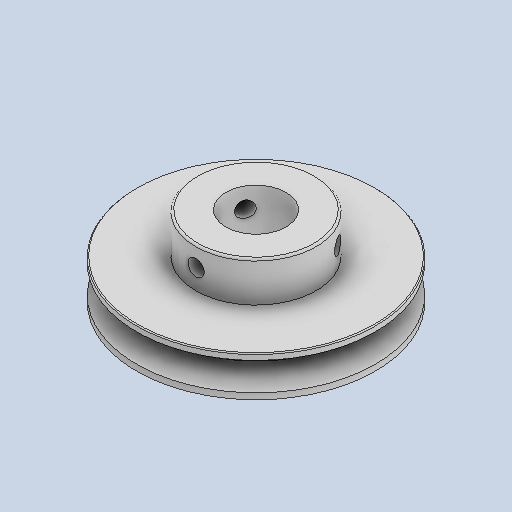
# Autodesk Inventor part: Шкив 119 мм
Saved by Autodesk Inventor 2025 (Build 290162010, 162A)
## iProperties
Created: 2024-04-08
Part Number: Шкив 119 мм
Material: Generic
Document SubType Name: Modeling
Designer: pokla
Density: 1 g/cm^3
Appearance: Default
Author: pokla
Autodesk Inventor part; units mm, degrees
ref_plane "YZ Plane" through (0, 0, 0) normal (1, 0, 0) x (0, 1, 0)
ref_plane "XZ Plane" through (0, 0, 0) normal (0, 1, 0) x (-1, 0, 0)
ref_plane "XY Plane" through (0, 0, 0) normal (0, 0, 1) x (1, 0, 0)
sketch "Sketch1" plane through (0, 0, 0) normal (1, 0, 0) x (0, 1, 0)
  line L0 (0, -15) -> (40, -15)
  line L1 (40, -15) -> (40, -30)
  line L2 (40, -30) -> (20, -30)
  line L3 (20, -30) -> (20, -59.5)
  line L4 (20, -59.5) -> (17, -59.5)
  line L5 (17, -59.5) -> (12.5, -46.5)
  line L6 (12.5, -46.5) -> (7.5, -46.5)
  line L7 (3, -59.5) -> (0, -59.5)
  line L8 (0, -59.5) -> (0, -15)
  line L9 (7.5, -46.5) -> (3, -59.5)
  line L10 (-8, 0) -> (48, 0) projected
  point P0 (0, 0)
  point P1 (0, -37.25)
  dimension "d0" = 15
  dimension "d1" = 59.5
  dimension "d2" = 40
  dimension "d3" = 20
  dimension "d4" = 5
  dimension "d5" = 3
  dimension "d7" = 46.5
  dimension "d8" = 15
  constraints: 20 end point, 5 perpendicular, 2 equal length, 2 point on line, 1 horizontal, 1 midpoint, 1 parallel, 1 vertical alignment
  measures "d0" distance of point (0, 0) L0.start
  measures "d1" distance of L7.end point (0, 0)
  measures "d2" distance of L0.start L0.end
  measures "d3" distance between parallel lines of L8 L3
  measures "d4" distance of L5.end L6.end
  measures "d5" distance of L7.start L7.end
  measures "d7" distance from line of point (0, 0) L6
  measures "d8" distance of L0.end L1.end
revolve "Revolution1" add sketch "Sketch1" angle 360 about axis through (0, -10, 0) along (0, 1, 0)
fillet "Fillet1" radius 1 1 edges at (0, 40, 30)
fillet "Fillet2" radius 0.5 1 edges at (0, 20, 59.5)
sketch "Sketch3" plane through (0, 0, 0) normal (0, 0, 1) x (1, 0, 0)
  line L0 (-29, 40) -> (29, 40) projected
  line L1 (-29, 30) -> (29, 30)
  circle A0 centre (0, 30) radius 4
  point P0 (0, 0)
  dimension "d17" = 10
  dimension "d18" = 8
  constraints: 2 end point, 1 centre point, 1 midpoint, 1 parallel, 1 vertical alignment
  measures "d17" distance between parallel lines of L0 L1
  measures "d18" diameter of A0
extrude "Extrusion2" cut sketch "Sketch3" along normal through all
pattern_circular "Circular Pattern1" count 3 over 360 about axis through (0, -10, 0) along (0, 1, 0) of "Extrusion2"
body "Solid1"
